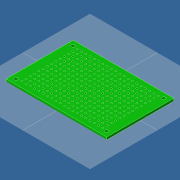
# Autodesk Inventor part: PCB_60x40
Saved by Autodesk Inventor 2016 SP2 (Build 200236200, 236)
## iProperties
Created: 2017-11-11
Part Number: PCB_60x40
Material: Generisch
Document SubType Name: Modeling
Designer: User
Density: 1 g/cm^3
Appearance: Dunkelgrün
Author: User
Autodesk Inventor part; units mm, degrees
ref_plane "YZ Plane" through (0, 0, 0) normal (1, 0, 0) x (0, 1, 0)
ref_plane "XZ Plane" through (0, 0, 0) normal (0, 1, 0) x (-1, 0, 0)
ref_plane "XY Plane" through (0, 0, 0) normal (0, 0, 1) x (1, 0, 0)
sketch "Skizze1" plane through (0, 0, 0) normal (0, 0, 1) x (1, 0, 0)
  line L0 (30, -20) -> (-30, -20)
  line L1 (-30, -20) -> (-30, 20)
  line L2 (-30, 20) -> (30, 20)
  line L3 (30, 20) -> (30, -20)
  line L4 (30, -20) -> (-30, 20) construction
  line L5 (-30, -20) -> (30, 20) construction
  circle A0 centre (-27, 17) radius 1
  circle A1 centre (-27, -17) radius 1
  circle A2 centre (27, 17) radius 1
  circle A3 centre (27, -17) radius 1
  line L6 (-42, 0) -> (42, 0) construction
  line L7 (0, -28) -> (0, 28) construction
  point P0 (0, 0)
  dimension "d0" = 60
  dimension "d1" = 40
  dimension "d45" = 2
  dimension "d46" = 54
  dimension "d47" = 34
  constraints: 12 end point, 4 centre point, 3 equal radius, 2 horizontal alignment, 2 midpoint, 2 parallel, 2 symmetric about line, 2 vertical alignment, 1 horizontal, 1 perpendicular
  measures "d0" distance of L1.end L2.end
  measures "d1" distance of L0.end L1.end
  measures "d45" diameter of A0
  measures "d46" distance of A2.centre A0.centre
  measures "d47" distance of A3.centre A2.centre
extrude "Extrusion1" add sketch "Skizze1" along normal blind 1.5 contours L0 L1 L2 L3 | A0 | A1 | A2 | A3
sketch "Skizze2" plane through (0, 0, 1.5) normal (0, 0, 1) x (1, 0, 0)
  line L0 (-42, 0) -> (42, 0) projected
  line L1 (0, -28) -> (0, 28) projected
  point P0 (0, 0)
  point P1 (-1.27, 1.27)
  point P2 (1.27, 1.27)
  point P3 (1.27, -1.27)
  point P4 (-1.27, -1.27)
  point P5 (-1.27, 3.81)
  point P6 (-1.27, 6.35)
  point P7 (-1.27, 8.89)
  point P8 (-1.27, 11.43)
  point P9 (-1.27, 13.97)
  point P10 (-1.27, 16.51)
  point P11 (-3.81, 1.27)
  point P12 (-3.81, 3.81)
  point P13 (-3.81, 6.35)
  point P14 (-3.81, 8.89)
  point P15 (-3.81, 11.43)
  point P16 (-3.81, 13.97)
  point P17 (-3.81, 16.51)
  point P18 (-6.35, 1.27)
  point P19 (-6.35, 3.81)
  point P20 (-6.35, 6.35)
  point P21 (-6.35, 8.89)
  point P22 (-6.35, 11.43)
  point P23 (-6.35, 13.97)
  point P24 (-6.35, 16.51)
  point P25 (-8.89, 1.27)
  point P26 (-8.89, 3.81)
  point P27 (-8.89, 6.35)
  point P28 (-8.89, 8.89)
  point P29 (-8.89, 11.43)
  point P30 (-8.89, 13.97)
  point P31 (-8.89, 16.51)
  point P32 (-11.43, 1.27)
  point P33 (-11.43, 3.81)
  point P34 (-11.43, 6.35)
  point P35 (-11.43, 8.89)
  point P36 (-11.43, 11.43)
  point P37 (-11.43, 13.97)
  point P38 (-11.43, 16.51)
  point P39 (-13.97, 1.27)
  point P40 (-13.97, 3.81)
  point P41 (-13.97, 6.35)
  point P42 (-13.97, 8.89)
  point P43 (-13.97, 11.43)
  point P44 (-13.97, 13.97)
  point P45 (-13.97, 16.51)
  point P46 (-16.51, 1.27)
  point P47 (-16.51, 3.81)
  point P48 (-16.51, 6.35)
  point P49 (-16.51, 8.89)
  point P50 (-16.51, 11.43)
  point P51 (-16.51, 13.97)
  point P52 (-16.51, 16.51)
  point P53 (-19.05, 1.27)
  point P54 (-19.05, 3.81)
  point P55 (-19.05, 6.35)
  point P56 (-19.05, 8.89)
  point P57 (-19.05, 11.43)
  point P58 (-19.05, 13.97)
  point P59 (-19.05, 16.51)
  point P60 (-21.59, 1.27)
  point P61 (-21.59, 3.81)
  point P62 (-21.59, 6.35)
  point P63 (-21.59, 8.89)
  point P64 (-21.59, 11.43)
  point P65 (-21.59, 13.97)
  point P66 (-21.59, 16.51)
  point P67 (-24.13, 1.27)
  point P68 (-24.13, 3.81)
  point P69 (-24.13, 6.35)
  point P70 (-24.13, 8.89)
  point P71 (-24.13, 11.43)
  point P72 (-24.13, 13.97)
  point P73 (-24.13, 16.51)
  point P74 (3.81, 1.27)
  point P75 (6.35, 1.27)
  point P76 (8.89, 1.27)
  point P77 (11.43, 1.27)
  point P78 (13.97, 1.27)
  point P79 (16.51, 1.27)
  point P80 (19.05, 1.27)
  point P81 (21.59, 1.27)
  point P82 (24.13, 1.27)
  point P83 (1.27, 3.81)
  point P84 (3.81, 3.81)
  point P85 (6.35, 3.81)
  point P86 (8.89, 3.81)
  point P87 (11.43, 3.81)
  point P88 (13.97, 3.81)
  point P89 (16.51, 3.81)
  point P90 (19.05, 3.81)
  point P91 (21.59, 3.81)
  point P92 (24.13, 3.81)
  point P93 (1.27, 6.35)
  point P94 (3.81, 6.35)
  point P95 (6.35, 6.35)
  point P96 (8.89, 6.35)
  point P97 (11.43, 6.35)
  point P98 (13.97, 6.35)
  point P99 (16.51, 6.35)
  point P100 (19.05, 6.35)
  point P101 (21.59, 6.35)
  point P102 (24.13, 6.35)
  point P103 (1.27, 8.89)
  point P104 (3.81, 8.89)
  point P105 (6.35, 8.89)
  point P106 (8.89, 8.89)
  point P107 (11.43, 8.89)
  point P108 (13.97, 8.89)
  point P109 (16.51, 8.89)
  point P110 (19.05, 8.89)
  point P111 (21.59, 8.89)
  point P112 (24.13, 8.89)
  point P113 (1.27, 11.43)
  point P114 (3.81, 11.43)
  point P115 (6.35, 11.43)
  point P116 (8.89, 11.43)
  point P117 (11.43, 11.43)
  point P118 (13.97, 11.43)
  point P119 (16.51, 11.43)
  point P120 (19.05, 11.43)
  point P121 (21.59, 11.43)
  point P122 (24.13, 11.43)
  point P123 (1.27, 13.97)
  point P124 (3.81, 13.97)
  point P125 (6.35, 13.97)
  point P126 (8.89, 13.97)
  point P127 (11.43, 13.97)
  point P128 (13.97, 13.97)
  point P129 (16.51, 13.97)
  point P130 (19.05, 13.97)
  point P131 (21.59, 13.97)
  point P132 (24.13, 13.97)
  point P133 (1.27, 16.51)
  point P134 (3.81, 16.51)
  point P135 (6.35, 16.51)
  point P136 (8.89, 16.51)
  point P137 (11.43, 16.51)
  point P138 (13.97, 16.51)
  point P139 (16.51, 16.51)
  point P140 (19.05, 16.51)
  point P141 (21.59, 16.51)
  point P142 (24.13, 16.51)
  point P143 (-1.27, -3.81)
  point P144 (-1.27, -6.35)
  point P145 (-1.27, -8.89)
  point P146 (-1.27, -11.43)
  point P147 (-1.27, -13.97)
  point P148 (-1.27, -16.51)
  point P149 (-3.81, -1.27)
  point P150 (-3.81, -3.81)
  point P151 (-3.81, -6.35)
  point P152 (-3.81, -8.89)
  point P153 (-3.81, -11.43)
  point P154 (-3.81, -13.97)
  point P155 (-3.81, -16.51)
  point P156 (-6.35, -1.27)
  point P157 (-6.35, -3.81)
  point P158 (-6.35, -6.35)
  point P159 (-6.35, -8.89)
  point P160 (-6.35, -11.43)
  point P161 (-6.35, -13.97)
  point P162 (-6.35, -16.51)
  point P163 (-8.89, -1.27)
  point P164 (-8.89, -3.81)
  point P165 (-8.89, -6.35)
  point P166 (-8.89, -8.89)
  point P167 (-8.89, -11.43)
  point P168 (-8.89, -13.97)
  point P169 (-8.89, -16.51)
  point P170 (-11.43, -1.27)
  point P171 (-11.43, -3.81)
  point P172 (-11.43, -6.35)
  point P173 (-11.43, -8.89)
  point P174 (-11.43, -11.43)
  point P175 (-11.43, -13.97)
  point P176 (-11.43, -16.51)
  point P177 (-13.97, -1.27)
  point P178 (-13.97, -3.81)
  point P179 (-13.97, -6.35)
  point P180 (-13.97, -8.89)
  point P181 (-13.97, -11.43)
  point P182 (-13.97, -13.97)
  point P183 (-13.97, -16.51)
  point P184 (-16.51, -1.27)
  point P185 (-16.51, -3.81)
  point P186 (-16.51, -6.35)
  point P187 (-16.51, -8.89)
  point P188 (-16.51, -11.43)
  point P189 (-16.51, -13.97)
  point P190 (-16.51, -16.51)
  point P191 (-19.05, -1.27)
  point P192 (-19.05, -3.81)
  point P193 (-19.05, -6.35)
  point P194 (-19.05, -8.89)
  point P195 (-19.05, -11.43)
  point P196 (-19.05, -13.97)
  point P197 (-19.05, -16.51)
  point P198 (-21.59, -1.27)
  point P199 (-21.59, -3.81)
  dimension "d4" = 2.54
  dimension "d5" = 2.54
  dimension "d8" = 2.54
  dimension "d11" = 2.54
  dimension "d16" = 2.54
  dimension "d19" = 2.54
  dimension "d24" = 2.54
  dimension "d27" = 2.54
  dimension "d32" = 2.54
  dimension "d35" = 2.54
  constraints: 4 horizontal, 4 vertical, 2 horizontal alignment, 2 symmetric about line, 2 vertical alignment, 276 other
  measures "d4" distance of point (1.27, 1.27) point (-1.27, 1.27)
  measures "d5" distance of point (-1.27, -1.27) point (-1.27, 1.27)
  measures "d8" distance of point (-1.27, 1.27) point (-1.27, 3.81)
  measures "d11" distance of point (-1.27, 1.27) point (-3.81, 1.27)
  measures "d16" distance of point (1.27, 1.27) point (3.81, 1.27)
  measures "d19" distance of point (1.27, 1.27) point (1.27, 3.81)
  measures "d24" distance of point (-1.27, -1.27) point (-1.27, -3.81)
  measures "d27" distance of point (-1.27, -1.27) point (-3.81, -1.27)
  measures "d32" distance of point (1.27, -1.27) point (1.27, -3.81)
  measures "d35" distance of point (1.27, -1.27) point (3.81, -1.27)
hole "Bohrung1" at (-1.27, 1.27, 1.5) at (1.27, 1.27, 1.5) at (1.27, -1.27, 1.5) at (-1.27, -1.27, 1.5) at (-1.27, 3.81, 1.5) at (-1.27, 6.35, 1.5) at (-1.27, 8.89, 1.5) at (-1.27, 11.43, 1.5) at (-1.27, 13.97, 1.5) at (-1.27, 16.51, 1.5) at (-3.81, 1.27, 1.5) at (-3.81, 3.81, 1.5) at (-3.81, 6.35, 1.5) at (-3.81, 8.89, 1.5) at (-3.81, 11.43, 1.5) at (-3.81, 13.97, 1.5) at (-3.81, 16.51, 1.5) at (-6.35, 1.27, 1.5) at (-6.35, 3.81, 1.5) at (-6.35, 6.35, 1.5) at (-6.35, 8.89, 1.5) at (-6.35, 11.43, 1.5) at (-6.35, 13.97, 1.5) at (-6.35, 16.51, 1.5) at (-8.89, 1.27, 1.5) at (-8.89, 3.81, 1.5) at (-8.89, 6.35, 1.5) at (-8.89, 8.89, 1.5) at (-8.89, 11.43, 1.5) at (-8.89, 13.97, 1.5) at (-8.89, 16.51, 1.5) at (-11.43, 1.27, 1.5) at (-11.43, 3.81, 1.5) at (-11.43, 6.35, 1.5) at (-11.43, 8.89, 1.5) at (-11.43, 11.43, 1.5) at (-11.43, 13.97, 1.5) at (-11.43, 16.51, 1.5) at (-13.97, 1.27, 1.5) at (-13.97, 3.81, 1.5) at (-13.97, 6.35, 1.5) at (-13.97, 8.89, 1.5) at (-13.97, 11.43, 1.5) at (-13.97, 13.97, 1.5) at (-13.97, 16.51, 1.5) at (-16.51, 1.27, 1.5) at (-16.51, 3.81, 1.5) at (-16.51, 6.35, 1.5) at (-16.51, 8.89, 1.5) at (-16.51, 11.43, 1.5) direction (0, 0, -1) diameter 1 end through all and at (-16.51, 13.97, 1.5) (-16.51, 16.51, 1.5) (-19.05, 1.27, 1.5) (-19.05, 3.81, 1.5) (-19.05, 6.35, 1.5) (-19.05, 8.89, 1.5) (-19.05, 11.43, 1.5) (-19.05, 13.97, 1.5) (-19.05, 16.51, 1.5) (-21.59, 1.27, 1.5) (-21.59, 3.81, 1.5) (-21.59, 6.35, 1.5) (-21.59, 8.89, 1.5) (-21.59, 11.43, 1.5) (-21.59, 13.97, 1.5) (-21.59, 16.51, 1.5) (-24.13, 1.27, 1.5) (-24.13, 3.81, 1.5) (-24.13, 6.35, 1.5) (-24.13, 8.89, 1.5) (-24.13, 11.43, 1.5) (-24.13, 13.97, 1.5) (-24.13, 16.51, 1.5) (3.81, 1.27, 1.5) (6.35, 1.27, 1.5) (8.89, 1.27, 1.5) (11.43, 1.27, 1.5) (13.97, 1.27, 1.5) (16.51, 1.27, 1.5) (19.05, 1.27, 1.5) (21.59, 1.27, 1.5) (24.13, 1.27, 1.5) (1.27, 3.81, 1.5) (3.81, 3.81, 1.5) (6.35, 3.81, 1.5) (8.89, 3.81, 1.5) (11.43, 3.81, 1.5) (13.97, 3.81, 1.5) (16.51, 3.81, 1.5) (19.05, 3.81, 1.5) (21.59, 3.81, 1.5) (24.13, 3.81, 1.5) (1.27, 6.35, 1.5) (3.81, 6.35, 1.5) (6.35, 6.35, 1.5) (8.89, 6.35, 1.5) (11.43, 6.35, 1.5) (13.97, 6.35, 1.5) (16.51, 6.35, 1.5) (19.05, 6.35, 1.5) (21.59, 6.35, 1.5) (24.13, 6.35, 1.5) (1.27, 8.89, 1.5) (3.81, 8.89, 1.5) (6.35, 8.89, 1.5) (8.89, 8.89, 1.5) (11.43, 8.89, 1.5) (13.97, 8.89, 1.5) (16.51, 8.89, 1.5) (19.05, 8.89, 1.5) (21.59, 8.89, 1.5) (24.13, 8.89, 1.5) (1.27, 11.43, 1.5) (3.81, 11.43, 1.5) (6.35, 11.43, 1.5) (8.89, 11.43, 1.5) (11.43, 11.43, 1.5) (13.97, 11.43, 1.5) (16.51, 11.43, 1.5) (19.05, 11.43, 1.5) (21.59, 11.43, 1.5) (24.13, 11.43, 1.5) (1.27, 13.97, 1.5) (3.81, 13.97, 1.5) (6.35, 13.97, 1.5) (8.89, 13.97, 1.5) (11.43, 13.97, 1.5) (13.97, 13.97, 1.5) (16.51, 13.97, 1.5) (19.05, 13.97, 1.5) (21.59, 13.97, 1.5) (24.13, 13.97, 1.5) (1.27, 16.51, 1.5) (3.81, 16.51, 1.5) (6.35, 16.51, 1.5) (8.89, 16.51, 1.5) (11.43, 16.51, 1.5) (13.97, 16.51, 1.5) (16.51, 16.51, 1.5) (19.05, 16.51, 1.5) (21.59, 16.51, 1.5) (24.13, 16.51, 1.5) (-1.27, -3.81, 1.5) (-1.27, -6.35, 1.5) (-1.27, -8.89, 1.5) (-1.27, -11.43, 1.5) (-1.27, -13.97, 1.5) (-1.27, -16.51, 1.5) (-3.81, -1.27, 1.5) (-3.81, -3.81, 1.5) (-3.81, -6.35, 1.5) (-3.81, -8.89, 1.5) (-3.81, -11.43, 1.5) (-3.81, -13.97, 1.5) (-3.81, -16.51, 1.5) (-6.35, -1.27, 1.5) (-6.35, -3.81, 1.5) (-6.35, -6.35, 1.5) (-6.35, -8.89, 1.5) (-6.35, -11.43, 1.5) (-6.35, -13.97, 1.5) (-6.35, -16.51, 1.5) (-8.89, -1.27, 1.5) (-8.89, -3.81, 1.5) (-8.89, -6.35, 1.5) (-8.89, -8.89, 1.5) (-8.89, -11.43, 1.5) (-8.89, -13.97, 1.5) (-8.89, -16.51, 1.5) (-11.43, -1.27, 1.5) (-11.43, -3.81, 1.5) (-11.43, -6.35, 1.5) (-11.43, -8.89, 1.5) (-11.43, -11.43, 1.5) (-11.43, -13.97, 1.5) (-11.43, -16.51, 1.5) (-13.97, -1.27, 1.5) (-13.97, -3.81, 1.5) (-13.97, -6.35, 1.5) (-13.97, -8.89, 1.5) (-13.97, -11.43, 1.5) (-13.97, -13.97, 1.5) (-13.97, -16.51, 1.5) (-16.51, -1.27, 1.5) (-16.51, -3.81, 1.5) (-16.51, -6.35, 1.5) (-16.51, -8.89, 1.5) (-16.51, -11.43, 1.5) (-16.51, -13.97, 1.5) (-16.51, -16.51, 1.5) (-19.05, -1.27, 1.5) (-19.05, -3.81, 1.5) (-19.05, -6.35, 1.5) (-19.05, -8.89, 1.5) (-19.05, -11.43, 1.5) (-19.05, -13.97, 1.5) (-19.05, -16.51, 1.5) (-21.59, -1.27, 1.5) (-21.59, -3.81, 1.5) (-21.59, -6.35, 1.5) (-21.59, -8.89, 1.5) (-21.59, -11.43, 1.5) (-21.59, -13.97, 1.5) (-21.59, -16.51, 1.5) (-24.13, -1.27, 1.5) (-24.13, -3.81, 1.5) (-24.13, -6.35, 1.5) (-24.13, -8.89, 1.5) (-24.13, -11.43, 1.5) (-24.13, -13.97, 1.5) (-24.13, -16.51, 1.5) (1.27, -3.81, 1.5) (1.27, -6.35, 1.5) (1.27, -8.89, 1.5) (1.27, -11.43, 1.5) (1.27, -13.97, 1.5) (1.27, -16.51, 1.5) (3.81, -1.27, 1.5) (3.81, -3.81, 1.5) (3.81, -6.35, 1.5) (3.81, -8.89, 1.5) (3.81, -11.43, 1.5) (3.81, -13.97, 1.5) (3.81, -16.51, 1.5) (6.35, -1.27, 1.5) (6.35, -3.81, 1.5) (6.35, -6.35, 1.5) (6.35, -8.89, 1.5) (6.35, -11.43, 1.5) (6.35, -13.97, 1.5) (6.35, -16.51, 1.5) (8.89, -1.27, 1.5) (8.89, -3.81, 1.5) (8.89, -6.35, 1.5) (8.89, -8.89, 1.5) (8.89, -11.43, 1.5) (8.89, -13.97, 1.5) (8.89, -16.51, 1.5) (11.43, -1.27, 1.5) (11.43, -3.81, 1.5) (11.43, -6.35, 1.5) (11.43, -8.89, 1.5) (11.43, -11.43, 1.5) (11.43, -13.97, 1.5) (11.43, -16.51, 1.5) (13.97, -1.27, 1.5) (13.97, -3.81, 1.5) (13.97, -6.35, 1.5) (13.97, -8.89, 1.5) (13.97, -11.43, 1.5) (13.97, -13.97, 1.5) (13.97, -16.51, 1.5) (16.51, -1.27, 1.5) (16.51, -3.81, 1.5) (16.51, -6.35, 1.5) (16.51, -8.89, 1.5) (16.51, -11.43, 1.5) (16.51, -13.97, 1.5) (16.51, -16.51, 1.5) (19.05, -1.27, 1.5) (19.05, -3.81, 1.5) (19.05, -6.35, 1.5) (19.05, -8.89, 1.5) (19.05, -11.43, 1.5) (19.05, -13.97, 1.5) (19.05, -16.51, 1.5) (21.59, -1.27, 1.5) (21.59, -3.81, 1.5) (21.59, -6.35, 1.5) (21.59, -8.89, 1.5) (21.59, -11.43, 1.5) (21.59, -13.97, 1.5) (21.59, -16.51, 1.5) (24.13, -1.27, 1.5) (24.13, -3.81, 1.5) (24.13, -6.35, 1.5) (24.13, -8.89, 1.5) (24.13, -11.43, 1.5) (24.13, -13.97, 1.5) (24.13, -16.51, 1.5)
extrude "Extrusion2" cut sketch "Skizze1" along normal through all contours A0 | A1 | A2 | A3
